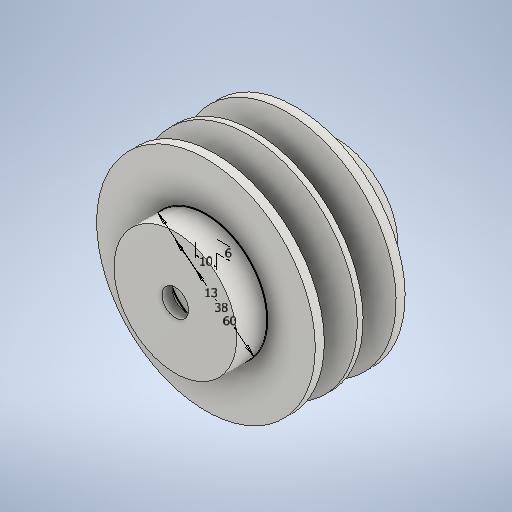
# Autodesk Inventor part: Grooved Pulley1
Saved by Autodesk Inventor 2025 (Build 290162000, 162)
## iProperties
CustomPartVersion: 1
Created: 2025-05-25
Part Number: Grooved Pulley1
Material: Steel
Document SubType Name: Modeling
Designer: Abdullah
Density: 1 g/cm^3
Appearance: Steel
Author: Abdullah
Autodesk Inventor part; units mm, degrees
ref_plane "YZ Plane" through (0, 0, 0) normal (1, 0, 0) x (0, 1, 0)
sketch "Main Sketch" plane through (0, 0, 0) normal (1, 0, 0) x (0, 1, 0)
  line L0 (0, 44) -> (53.5, 44)
  line L1 (53.5, 44) -> (53.5, 20.5701)
  line L2 (53.5, 20.5701) -> (36, 15.2198)
  line L3 (36, 15.2198) -> (36, 9.7802)
  line L4 (36, 9.7802) -> (53.5, 4.4299)
  line L5 (53.5, 4.4299) -> (53.5, 0)
  line L6 (53.5, 0) -> (0, 0)
  line L7 (50, 19.5) -> (50, 5.5) construction
  line L8 (36, 12.5) -> (50, 12.5) construction
  line L9 (53.5, 20.5701) -> (53.5, 4.4299)
  line L10 (0, -4) -> (0, 24) projected
  line L11 (0, 0) -> (0, 44)
  dimension "d0" = 14
  dimension "d1" = 34
  dimension "d2" = 3.5
  dimension "d6" = 44
  dimension "d21" = 100
  dimension "d25" = 17.5
  dimension "d27" = 12.5
  constraints: 22 end point, 5 perpendicular, 2 collinear, 2 midpoint, 2 point on line, 1 parallel
  measures "d0" distance of L7.start L7.end
  measures "d1" angle of L2 L4
  measures "d2" distance between parallel lines of L1 L7
  measures "d6" distance between parallel lines of L6 L0
  measures "d21" diameter of L7 L10
  measures "d25" distance between parallel lines of L3 L9
  measures "d27" distance between parallel lines of L6 L8
ref_plane "Belt Plane" through (0, 36, 12.5) normal (0, 0, 1) x (1, 0, 0)
revolve "Body" add sketch "Main Sketch" angle 360 about axis through (0, 0, -10) along (0, 0, 1)
revolve "Groove" cut sketch "Main Sketch" angle 360 about axis through (0, 0, -10) along (0, 0, 1) contours L9 L4 L3 L2
fillet "Fillet External" [suppressed]
fillet "Fillet Internal" [suppressed]
pattern_linear "Groove Pattern" count 2 spacing 19 along (0, 0, 1) of "Groove"
sketch "Sketch2" plane through (0, 0, 44) normal (0, 0, 1) x (1, 0, 0)
  circle A0 centre (0, 0) radius 19
  circle A1 centre (0, 0) radius 30
  line L0 (-5, 22) -> (5, 22)
  line L1 (5, 22) -> (5, 16)
  line L2 (5, 16) -> (-5, 16)
  line L3 (-5, 16) -> (-5, 22)
  line L4 (-5, 22) -> (5, 16) construction
  line L5 (5, 22) -> (-5, 16) construction
  circle A2 centre (0, 0) radius 6.5
  point P0 (0, 19)
  point P1 (5, 18.3303)
  point P2 (-5, 18.3303)
  dimension "d28" = 38
  dimension "d29" = 60
  dimension "d30" = 10
  dimension "d31" = 6
  dimension "d47" = 13
  constraints: 12 end point, 3 coincident, 2 centre point, 2 midpoint, 2 parallel, 1 horizontal, 1 perpendicular, 3 other
  measures "d29" diameter of A1
  measures "d30" distance of L1.end L2.end
  measures "d31" distance of L0.end L1.end
  measures "d47" diameter of A2
extrude "Extrusion1" add sketch "Sketch2" against normal blind 20 from surface at -44 contours A1
ref_plane "Work Plane2" through (0, 30, 44) normal (0, 1, 0) x (-1, 0, 0)
sketch "Sketch3" plane through (0, 30, 44) normal (0, 1, 0) x (-1, 0, 0)
  line L0 (0, -44) -> (0, -64)
  line L1 (30, -64) -> (-30, -64) projected
  circle A0 centre (0, -52.2223) radius 5
  dimension "d34" = 10
  constraints: 2 end point, 1 centre point, 1 coincident, 1 midpoint, 1 point on line
  measures "d34" diameter of A0
hole "Hole1" at (0, 30, -8.2223) direction (0, -1, 0) diameter 8.376 depth 27.3 tip angle 118 thread size "M10x1.5" class "6H" standard "ISO Metric profile"
extrude "Extrusion2" cut sketch "Sketch2" against normal through all contours A0 L3 L2 L1 | L1 L2 L3 A0 | A0 L3 L0 L1 | A2
pattern_circular "Circular Pattern1" count 2 over 90 about axis through (0, 0, 44) along (0, 0, 1) of "Hole1"
extrude "Extrusion3" add sketch "Sketch2" along normal blind 10 separate body contours A1
sketch "Sketch4" plane through (0, 0, 54) normal (0, 0, 1) x (1, 0, 0)
  circle A0 centre (0, 0) radius 30
  arc A1 (-5, 18.3303) -> (5, 18.3303) centre (0, 0) ccw projected
  circle A2 centre (0, 0) radius 6.5
  dimension "d50" = 13
  constraints: 2 centre point, 2 coincident
  measures "d50" diameter of A2
extrude "Extrusion4" add sketch "Sketch4" along normal blind 5 bodies 2
equation "\"d0\" = da_Bw"
equation "\"d1\" = da_Alfa"
equation "\"d2\" = da_c"
equation "\"d21\" = da_Dw"
equation "\"d25\" = da_Hd"
equation "\"d27\" = da_Se"
equation "\"da_r1\" = 0"
equation "\"da_r2\" = 0"
equation "\"d18\" = da_Sg"
equation "\"d5\" = da_Se"
equation "\"da_Bw\" = 14"
equation "\"da_Alfa\" = 34deg"
equation "\"da_c\" = 3.5"
equation "\"da_Dw\" = 100"
equation "\"da_Hd\" = 17.5"
equation "\"da_Se\" = 12.5"
equation "\"da_Sg\" = 19"
body "Solid1"
body "Solid2"
